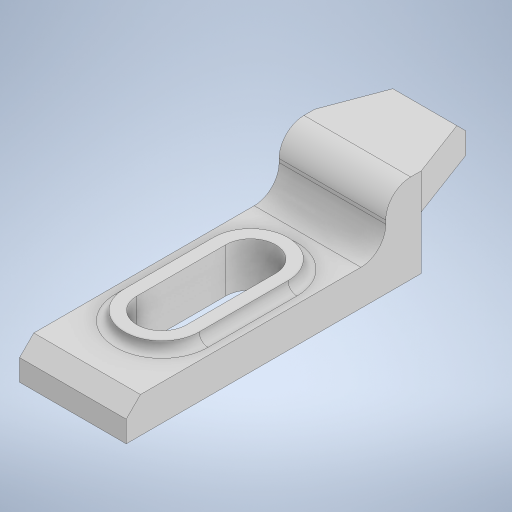
# Autodesk Inventor part: esercizio 040.20 03-02-2023
Saved by Autodesk Inventor 2023 (Build 270158000, 158)
## iProperties
Created: 2023-03-02
Part Number: esercizio 040.20 03-02-2023
Material: Generico
Document SubType Name: Modeling
Designer: Admin
Density: 1 g/cm^3
Appearance: Default
Author: Admin
Autodesk Inventor part; units mm, degrees
ref_plane "YZ Plane" through (0, 0, 0) normal (1, 0, 0) x (0, 1, 0)
ref_plane "XZ Plane" through (0, 0, 0) normal (0, 1, 0) x (-1, 0, 0)
ref_plane "XY Plane" through (0, 0, 0) normal (0, 0, 1) x (1, 0, 0)
sketch "Schizzo1" plane through (0, 0, 0) normal (0, 1, 0) x (-1, 0, 0)
  line L0 (0, 0) -> (0, -83)
  line L1 (30, 0) -> (0, 0)
  line L2 (30, -73) -> (0, -73)
  line L3 (30, 0) -> (30, -83)
  line L4 (30, -83) -> (0, -83)
  line L5 (15, 0) -> (15, -130.8498) construction
  line L6 (22.5, -103) -> (15, -103)
  line L7 (30, -83) -> (22.5, -103)
  line L8 (0, -83) -> (7.5, -103)
  line L9 (15, 0) -> (15, -25) construction
  line L10 (15, -25) -> (15, -50) construction
  line L11 (8, -25) -> (8, -50)
  line L12 (22, -50) -> (22, -25)
  arc A0 (22, -25) -> (8, -25) centre (15, -25) ccw
  arc A1 (8, -50) -> (22, -50) centre (15, -50) ccw
  line L13 (15, -25) -> (15, -50) construction
  line L14 (2, -25) -> (2, -50)
  line L15 (28, -50) -> (28, -25)
  arc A2 (28, -25) -> (2, -25) centre (15, -25) ccw
  arc A3 (2, -50) -> (28, -50) centre (15, -50) ccw
  line L16 (15, -103) -> (7.5, -103)
  point P0 (15, -37.5)
  point P1 (15, -37.5)
  dimension "d5" = 83
  dimension "d10" = 20
  dimension "d11" = 30
  dimension "d15" = 30
  dimension "d17" = 25
  dimension "d18" = 25
  dimension "d19" = 7.5
  dimension "d20" = 7.5
  constraints: 38 end point, 8 point on circle, 8 tangent, 4 centre point, 4 parallel, 4 point on line, 4 vertical, 3 midpoint, 2 horizontal, 1 perpendicular
  measures "d5" distance between parallel lines of L1 L4
  measures "d10" distance between parallel lines of L4 L6
  measures "d11" distance between parallel lines of L6 L2
  measures "d15" distance of L1.start L0.start
  measures "d17" distance from line of L12.end L1
  measures "d18" distance of L11.start L11.end
  measures "d19" distance of L6.start L6.end
  measures "d20" distance of L6.end L8.end
extrude "Estrusione1" add sketch "Schizzo1" along normal blind 10 contours L1 L3 L2 L0
extrude "Estrusione2" add sketch "Schizzo1" along normal blind 12.5 contours A2 L15 A3 L14
extrude "Estrusione3" add sketch "Schizzo1" along normal blind 25 contours L2 L3 L4 L0 | L4 L7 L6 L16 L8
extrude "Estrusione4" cut sketch "Schizzo1" along normal blind 15 contours L4 L7 L6 L16 L8
fillet "Raccordo1" radius 7 2 edges at (-15, 25, -73) (-15, 10, -73)
fillet "Raccordo2" radius 2.5 4 edges at (-2, 12.5, -37.5) (-15, 12.5, -63) (-28, 12.5, -37.5) (-15, 12.5, -12) inverted yes
chamfer "Smusso1" distance 4 angle 45 2 edges at (-15, 25, -103) (-15, 10, 0)
